Autodesk Fusion 360 part; units mm, degrees
(part 8 of 8)
  spline S51 degree 5 poles (-35.2993, -22.9766) (-35.2936, -22.9816) (-35.2824, -22.9916) (-35.2655, -23.0066) (-35.2429, -23.0265) (-35.2146, -23.0512) (-35.1862, -23.0757) (-35.1578, -23.1001) (-35.1293, -23.1243) (-35.1008, -23.1484) (-35.0721, -23.1723) (-35.0434, -23.196) (-35.0147, -23.2196) (-34.9858, -23.243) (-34.9569, -23.2663) (-34.9279, -23.2894) (-34.8989, -23.3123) (-34.8698, -23.3351) (-34.8406, -23.3577) (-34.8114, -23.3802) (-34.7821, -23.4024) (-34.7527, -23.4245) (-34.7233, -23.4465) (-34.6938, -23.4682) (-34.6642, -23.4898) (-34.6346, -23.5112) (-34.6049, -23.5324) (-34.5751, -23.5535) (-34.5453, -23.5744) (-34.5154, -23.595) (-34.4855, -23.6155) (-34.4554, -23.6358) (-34.4253, -23.656) (-34.3952, -23.6759) (-34.365, -23.6956) (-34.3347, -23.7152) (-34.3043, -23.7345) (-34.2739, -23.7537) (-34.2434, -23.7726) (-34.2129, -23.7914) (-34.1822, -23.8099) (-34.1516, -23.8283) (-34.1208, -23.8464) (-34.09, -23.8643) (-34.0591, -23.8819) (-34.0282, -23.8994) (-33.9971, -23.9166) (-33.9661, -23.9336) (-33.9349, -23.9504) (-33.9037, -23.967) (-33.8724, -23.9833) (-33.8411, -23.9993) (-33.8096, -24.0151) (-33.7781, -24.0306) (-33.7465, -24.0458) (-33.7149, -24.0608) (-33.6832, -24.0755) (-33.6514, -24.09) (-33.6196, -24.1043) (-33.5877, -24.1182) (-33.5557, -24.1318) (-33.5236, -24.1449) (-33.4914, -24.1577) (-33.4591, -24.17) (-33.4267, -24.1819) (-33.3942, -24.1935) (-33.3617, -24.2049) (-33.3292, -24.2161) (-33.2966, -24.227) (-33.2639, -24.2373) (-33.231, -24.2466) (-33.2044, -24.2531) (-33.1843, -24.2573) (-33.1709, -24.2598) (-33.1641, -24.2609) knots -1 -1 -1 -1 -1 -1 -0.98571429 -0.97142857 -0.95714286 -0.94285714 -0.92857143 -0.91428571 -0.9 -0.88571429 -0.87142857 -0.85714286 -0.84285714 -0.82857143 -0.81428571 -0.8 -0.78571429 -0.77142857 -0.75714286 -0.74285714 -0.72857143 -0.71428571 -0.7 -0.68571429 -0.67142857 -0.65714286 -0.64285714 -0.62857143 -0.61428571 -0.6 -0.58571429 -0.57142857 -0.55714286 -0.54285714 -0.52857143 -0.51428571 -0.5 -0.48571429 -0.47142857 -0.45714286 -0.44285714 -0.42857143 -0.41428571 -0.4 -0.38571429 -0.37142857 -0.35714286 -0.34285714 -0.32857143 -0.31428571 -0.3 -0.28571429 -0.27142857 -0.25714286 -0.24285714 -0.22857143 -0.21428571 -0.2 -0.18571429 -0.17142857 -0.15714286 -0.14285714 -0.12857143 -0.11428571 -0.1 -0.08571429 -0.07142857 -0.05714286 -0.04285714 -0.02857143 -0.01428571 0 0 0 0 0 0
  line L51 (-33.1641, -24.2609) -> (-33.0602, -24.2787)
  arc A103 (-32.6491, -24.8397) -> (-33.0602, -24.2787) centre (-33.1444, -24.7715) ccw
  circle A104 centre (-17.3506, -26.9445) radius 2.7
  circle A105 centre (-17.3506, -26.9445) radius 2.7
  circle A106 centre (-17.3506, -26.9445) radius 2.7
  circle A107 centre (-17.3506, -26.9445) radius 4.25
  dimension "d37" = 8.5
  constraint concentric A0 A105
  constraint concentric A105 A106
  constraint concentric A105 A107
  measures "d37" diameter of A107
extrude "Extrude3" add sketch "Sketch1 (2)" along normal blind 9 contours A107 sketch seen with x (1, 0, 0) y (0, 1, 0) z (0, 0, 1) at (-17.3506, -26.9445, 0) in component "Spur Gear (26 teeth)"
hole "Hole1" at (0, 4.25, 12.9882) direction (0, -1, 0) diameter 3 depth 3 tip angle 118 in component "Spur Gear (26 teeth)"
hole "Hole2" at (-4.25, 0, 12.9257) direction (1, 0, 0) diameter 2 depth 3 tip angle 118 in component "Spur Gear (26 teeth)"
hole "Hole3" at (0, -4.25, 12.2277) direction (0, 1, 0) diameter 2.5 depth 3 tip angle 118 in component "Spur Gear (26 teeth)"
hole "Hole4" at (4.25, 0, 13.2547) direction (-1, 0, 0) diameter 2.75 depth 3 tip angle 118 in component "Spur Gear (26 teeth)"
sketch "Sketch2 (2)" plane through (0, 0, 0) normal (0, 1, 0) x (1, 0, 0)
  circle A0 centre (-38.9137, -5.4395) radius 4.5
  circle A1 centre (-38.9137, -5.4395) radius 6.5
  dimension "d52" = 9
  dimension "d53" = 13
  constraint concentric A0 A1
  measures "d52" diameter of A0
  measures "d53" diameter of A1
combine "Combine1" [no effect]
sketch "Sketch3 (2)" plane through (0, 0, 0) normal (1, 0, 0) x (0, 1, 0)
  line L0 (105.0534, -1.0193) -> (-2.1023, -1.0193)
  circle A0 centre (96.2618, -1.0193) radius 1.5
  circle A1 centre (83.5203, -1.0193) radius 1.375
  circle A2 centre (73.2634, -1.0193) radius 1.25
  circle A3 centre (64.1533, -1.0193) radius 1
  circle A4 centre (54.852, -1.0193) radius 1.5
  circle A5 centre (47.2708, -1.0193) radius 1.55
  circle A6 centre (39.3074, -1.0193) radius 1.375
  circle A7 centre (30.7706, -1.0193) radius 1.25
  circle A8 centre (22.0427, -1.0193) radius 1
  circle A9 centre (12.1681, -1.0193) radius 1.5
  circle A10 centre (4.0136, -1.0193) radius 1.5
  dimension "d56" = 3
  dimension "d57" = 2.75
  dimension "d58" = 2.5
  dimension "d59" = 2
  dimension "d60" = 3
  dimension "d61" = 3.1
  dimension "d62" = 2.75
  dimension "d63" = 2.5
  dimension "d64" = 2
  dimension "d65" = 3
  dimension "d66" = 3
  constraint horizontal L0
  constraint coincident L0 A0.centre
  constraint coincident L0 A1.centre
  constraint coincident L0 A2.centre
  constraint coincident L0 A3.centre
  constraint coincident L0 A4.centre
  constraint coincident L0 A5.centre
  constraint coincident L0 A6.centre
  constraint coincident L0 A7.centre
  constraint coincident L0 A8.centre
  constraint coincident L0 A9.centre
  constraint coincident L0 A10.centre
  measures "d56" diameter of A0
  measures "d57" diameter of A1
  measures "d58" diameter of A2
  measures "d59" diameter of A3
  measures "d60" diameter of A4
  measures "d61" diameter of A5
  measures "d62" diameter of A6
  measures "d63" diameter of A7
  measures "d64" diameter of A8
  measures "d65" diameter of A9
  measures "d66" diameter of A10
component "Spur Gear (26 teeth)" placed x (1, 0, 0) y (0, 1, 0) z (0, 0, 1) at (17.3506, 26.9445, -4)
